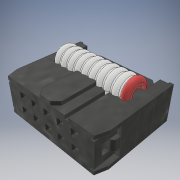
# Autodesk Inventor part: Connector-2x5
Saved by Autodesk Inventor 2018 (Build 220112000, 112)
## iProperties
Created: 2021-02-20
Part Number: Connector-2x5
Material: Všeobecné
Document SubType Name: Modeling
Designer: Jozko Mrkvicka
Density: 1 g/cm^3
Appearance: Výchozí
Author: Jozko Mrkvicka
Autodesk Inventor part; units mm, degrees
sketch "Náčrt1" plane through (0, 0, 0) normal (0, 1, 0) x (-1, 0, 0)
  line L0 (3.175, 8.89) -> (-3.175, 8.89)
  line L1 (-3.175, 8.89) -> (-3.175, -8.89)
  line L2 (-3.175, -8.89) -> (3.175, -8.89)
  line L3 (3.175, -8.89) -> (3.175, 8.89)
  line L4 (3.175, 8.89) -> (-3.175, -8.89) construction
  line L5 (-3.175, 8.89) -> (3.175, -8.89) construction
  point P0 (0, 0)
  dimension "d0" = 6.35
  dimension "d1" = 17.78
  constraints: 12 end point, 2 midpoint, 2 parallel, 1 horizontal, 1 perpendicular
  measures "d0" distance of L2.end L1.end
  measures "d1" distance of L1.end L0.end
extrude "Vysunutí1" add sketch "Náčrt1" along normal blind 15.24
sketch "Náčrt2" plane through (0, 15.24, 0) normal (0, 1, 0) x (1, 0, 0)
  line L0 (-1.5875, -6.35) -> (-1.5875, 6.35)
  line L1 (-3.175, -6.985) -> (-1.5875, -6.985)
  line L2 (-1.5875, -6.985) -> (-1.5875, 6.985)
  line L3 (-1.5875, 6.985) -> (-3.175, 6.985)
  line L4 (-3.175, 6.985) -> (-3.175, -6.985)
  line L5 (-3.175, -6.985) -> (-1.5875, 6.985) construction
  line L6 (-1.5875, -6.985) -> (-3.175, 6.985) construction
  line L7 (3.175, -6.985) -> (1.5875, -6.985)
  line L8 (1.5875, -6.985) -> (1.5875, 6.985)
  line L9 (1.5875, 6.985) -> (3.175, 6.985)
  line L10 (3.175, 6.985) -> (3.175, -6.985)
  line L11 (3.175, -6.985) -> (1.5875, 6.985) construction
  line L12 (1.5875, -6.985) -> (3.175, 6.985) construction
  point P0 (0, 0)
  point P1 (-3.175, -6.35)
  point P2 (-2.3813, 0)
  point P3 (2.3813, 0)
  dimension "d18" = 13.97
  dimension "d19" = 13.97
  constraints: 26 end point, 4 midpoint, 4 parallel, 2 horizontal, 2 perpendicular
  measures "d18" distance of L2.end L1.end
  measures "d19" distance of L7.end L8.end
extrude "Vysunutí2" cut sketch "Náčrt2" against normal blind 5.08
sketch "Náčrt3" plane through (3.175, 0, 8.89) normal (1, 0, 0) x (0, 0, -1)
  line L0 (3.81, 15.24) -> (2.54, 13.97)
  line L1 (13.97, 15.24) -> (15.24, 13.97)
  line L2 (2.54, 13.97) -> (0.635, 13.97)
  line L3 (15.24, 13.97) -> (17.145, 13.97)
  line L4 (0.635, 13.97) -> (0.635, 14.2875)
  line L5 (0.635, 14.2875) -> (0, 14.2875)
  line L6 (17.145, 13.97) -> (17.145, 14.2875)
  line L7 (17.145, 14.2875) -> (17.78, 14.2875)
  line L8 (3.81, 15.24) -> (13.97, 15.24)
  line L9 (17.78, 14.2875) -> (17.78, 16.064)
  line L10 (17.78, 16.064) -> (0, 16.064)
  line L11 (0, 16.064) -> (0, 14.2875)
  line L12 (0.635, 13.97) -> (2.54, 13.97)
  line L13 (15.24, 13.97) -> (17.145, 13.97)
  point P0 (8.89, 0)
  point P1 (8.89, 15.24)
  constraints: 28 end point, 3 parallel, 3 perpendicular, 2 horizontal
extrude "Vysunutí3" cut sketch "Náčrt3" against normal up to surface (6.35 mm away)
sketch "Náčrt4" plane through (3.175, 0, 8.89) normal (1, 0, 0) x (0, 0, -1)
  line L0 (1.905, 6.985) -> (15.875, 6.985)
  line L1 (15.875, 6.985) -> (15.875, 11.43)
  line L2 (15.875, 11.43) -> (1.905, 11.43)
  line L3 (1.905, 11.43) -> (1.905, 6.985)
  point P0 (0, 0)
  point P1 (8.89, 0)
  constraints: 8 end point, 2 parallel, 1 horizontal, 1 perpendicular
extrude "Vysunutí4" cut sketch "Náčrt4" against normal up to surface (6.35 mm away)
sketch "Náčrt5" plane through (0, 0, 0) normal (0, -1, 0) x (1, 0, 0)
  line L0 (-3.175, 6.985) -> (-3.175, -6.985) projected
  line L1 (-1.27, 5.08) -> (1.27, 5.08)
  line L2 (1.27, 5.08) -> (1.27, -5.08)
  line L3 (0.9525, 4.7625) -> (1.5875, 4.7625)
  line L4 (1.5875, 4.7625) -> (1.5875, 5.3975)
  line L5 (1.5875, 5.3975) -> (0.9525, 5.3975)
  line L6 (0.9525, 5.3975) -> (0.9525, 4.7625)
  line L7 (0.9525, 4.7625) -> (1.5875, 5.3975) construction
  line L8 (1.5875, 4.7625) -> (0.9525, 5.3975) construction
  line L9 (1.5875, 2.2225) -> (1.5875, 2.8575)
  line L10 (1.5875, 2.8575) -> (0.9525, 2.8575)
  line L11 (0.9525, 2.2225) -> (1.5875, 2.2225)
  line L12 (0.9525, 2.8575) -> (0.9525, 2.2225)
  line L13 (1.5875, -0.3175) -> (1.5875, 0.3175)
  line L14 (1.5875, 0.3175) -> (0.9525, 0.3175)
  line L15 (0.9525, -0.3175) -> (1.5875, -0.3175)
  line L16 (0.9525, 0.3175) -> (0.9525, -0.3175)
  line L17 (1.5875, -2.8575) -> (1.5875, -2.2225)
  line L18 (1.5875, -2.2225) -> (0.9525, -2.2225)
  line L19 (0.9525, -2.8575) -> (1.5875, -2.8575)
  line L20 (0.9525, -2.2225) -> (0.9525, -2.8575)
  line L21 (1.5875, -5.3975) -> (1.5875, -4.7625)
  line L22 (1.5875, -4.7625) -> (0.9525, -4.7625)
  line L23 (0.9525, -5.3975) -> (1.5875, -5.3975)
  line L24 (0.9525, -4.7625) -> (0.9525, -5.3975)
  line L25 (-0.9525, 4.7625) -> (-0.9525, 5.3975)
  line L26 (-0.9525, 5.3975) -> (-1.5875, 5.3975)
  line L27 (-1.5875, 4.7625) -> (-0.9525, 4.7625)
  line L28 (-1.5875, 5.3975) -> (-1.5875, 4.7625)
  line L29 (-0.9525, 2.2225) -> (-0.9525, 2.8575)
  line L30 (-0.9525, 2.8575) -> (-1.5875, 2.8575)
  line L31 (-1.5875, 2.2225) -> (-0.9525, 2.2225)
  line L32 (-1.5875, 2.8575) -> (-1.5875, 2.2225)
  line L33 (-0.9525, -0.3175) -> (-0.9525, 0.3175)
  line L34 (-0.9525, 0.3175) -> (-1.5875, 0.3175)
  line L35 (-1.5875, -0.3175) -> (-0.9525, -0.3175)
  line L36 (-1.5875, 0.3175) -> (-1.5875, -0.3175)
  line L37 (-0.9525, -2.8575) -> (-0.9525, -2.2225)
  line L38 (-0.9525, -2.2225) -> (-1.5875, -2.2225)
  line L39 (-1.5875, -2.8575) -> (-0.9525, -2.8575)
  line L40 (-1.5875, -2.2225) -> (-1.5875, -2.8575)
  line L41 (-0.9525, -5.3975) -> (-0.9525, -4.7625)
  line L42 (-0.9525, -4.7625) -> (-1.5875, -4.7625)
  line L43 (-1.5875, -5.3975) -> (-0.9525, -5.3975)
  line L44 (-1.5875, -4.7625) -> (-1.5875, -5.3975)
  line L45 (1.5875, -4.7625) -> (1.5875, -2.8575)
  line L46 (3.175, -3.4925) -> (2.54, -3.4925)
  line L47 (2.54, -3.4925) -> (2.54, -4.1275)
  line L48 (2.54, -4.1275) -> (3.175, -4.1275)
  line L49 (3.175, -3.4925) -> (3.175, -4.1275)
  point P0 (0, 0)
  dimension "d30" = 2.54
  dimension "d33" = 2.54
  constraints: 98 end point, 4 horizontal, 3 parallel, 3 perpendicular, 2 midpoint, 2 vertical, 72 other
  measures "d30" distance of L3.end L9.start
  measures "d33" distance of L3.end L25.start
extrude "Vysunutí5" cut sketch "Náčrt5" against normal up to surface (6.985 mm away) contours L6 L5 L4 L3 L2 L1 | L1 L2 L3 L6 | L10 L9 L11 L2 | L2 L11 L12 L10 | L14 L13 L15 L2 | L2 L15 L16 L14 | L18 L17 L19 L2 | L2 L19 L20 L18 | L22 L21 L23 L24 | L27 L28 L26 L25 | L31 L32 L30 L29 | L35 L36 L34 L33 | L39 L40 L38 L37 | L43 L44 L42 L41 | L49 L48 L47 L46
chamfer "Zkosení1" distance 0.3175 angle 45 40 edges at (1.27, 0, 5.3975) (1.27, 0, 4.7625) (0.9525, 0, 5.08) (1.5875, 0, 5.08) (1.5875, 0, 2.54) (1.27, 0, 2.2225) (0.9525, 0, 2.54) (1.27, 0, 2.8575) (1.27, 0, 0.3175) (1.27, 0, -0.3175) (1.5875, 0, 0) (0.9525, 0, 0) (1.27, 0, -2.2225) (1.5875, 0, -2.54) (0.9525, 0, -2.54) (1.27, 0, -2.8575) (1.5875, 0, -5.08) (1.27, 0, -4.7625) (0.9525, 0, -5.08) (1.27, 0, -5.3975) (-0.9525, 0, -5.08) (-1.27, 0, -5.3975) (-1.5875, 0, -5.08) (-1.27, 0, -4.7625) (-1.5875, 0, -2.54) (-1.27, 0, -2.8575) (-0.9525, 0, -2.54) (-1.27, 0, -2.2225) (-1.5875, 0, 0) (-1.27, 0, -0.3175) (-0.9525, 0, 0) (-1.27, 0, 0.3175) (-1.5875, 0, 2.54) (-1.27, 0, 2.2225) (-0.9525, 0, 2.54) (-1.27, 0, 2.8575) (-1.5875, 0, 5.08) (-1.27, 0, 4.7625) (-0.9525, 0, 5.08) (-1.27, 0, 5.3975)
sketch "Náčrt6" plane through (3.175, 0, 8.89) normal (1, 0, 0) x (0, 0, -1)
  line L0 (10.795, 0.9525) -> (10.795, 6.985)
  line L1 (10.795, 6.985) -> (6.985, 6.985)
  line L2 (6.985, 6.985) -> (6.985, 0.9525)
  line L3 (10.795, 0.9525) -> (9.8425, 0)
  line L4 (6.985, 0.9525) -> (7.9375, 0)
  line L5 (7.9375, 0) -> (9.8425, 0)
  point P0 (8.89, 0)
  constraints: 12 end point, 1 parallel
extrude "Vysunutí6" add sketch "Náčrt6" along normal blind 0.635
sketch "Náčrt7" plane through (-3.175, 0, 8.89) normal (0, 0, 1) x (1, 0, 0)
  line L0 (0.635, 0) -> (5.715, 0)
  line L1 (5.715, 0) -> (5.715, 3.81)
  line L2 (0.635, 3.81) -> (0.635, 0)
  line L3 (4.1275, 3.81) -> (4.1275, 2.54)
  line L4 (4.1275, 2.54) -> (2.2225, 2.54)
  line L5 (2.2225, 2.54) -> (2.2225, 3.81)
  line L6 (5.715, 3.81) -> (4.1275, 3.81)
  line L7 (2.2225, 3.81) -> (0.635, 3.81)
  point P0 (3.175, 0)
  point P1 (3.175, 3.81)
  constraints: 16 end point, 4 parallel, 1 horizontal, 1 perpendicular
extrude "Vysunutí7" cut sketch "Náčrt7" against normal blind 1.27
sketch "Náčrt8" plane through (3.175, 0, -8.89) normal (0, 0, -1) x (-1, 0, 0)
  line L0 (0.635, 0) -> (5.715, 0) projected
  line L1 (0.635, 3.81) -> (0.635, 0) projected
  line L2 (2.2225, 3.81) -> (0.635, 3.81) projected
  line L3 (2.2225, 2.54) -> (2.2225, 3.81) projected
  line L4 (4.1275, 2.54) -> (2.2225, 2.54) projected
  line L5 (4.1275, 3.81) -> (4.1275, 2.54) projected
  line L6 (5.715, 3.81) -> (4.1275, 3.81) projected
  line L7 (5.715, 0) -> (5.715, 3.81) projected
extrude "Vysunutí8" cut sketch "Náčrt8" against normal blind 1.27
fillet "Zaoblení1" radius 0.635 2 edges at (0, 2.54, 8.89) (0, 2.54, -8.89)
sketch "Náčrt9" plane through (-3.175, 0, 7.62) normal (0, 0, 1) x (1, 0, 0)
  line L0 (5.715, 0) -> (0.635, 0) projected
  line L1 (4.1275, 3.81) -> (5.715, 3.81) projected
  line L2 (4.1275, 2.54) -> (4.1275, 3.81) projected
  line L3 (2.2225, 2.54) -> (4.1275, 2.54) projected
  line L4 (2.2225, 3.81) -> (2.2225, 2.54) projected
  line L5 (0.635, 3.81) -> (2.2225, 3.81) projected
  line L6 (5.715, 0) -> (5.3975, 0)
  line L7 (5.3975, 0) -> (5.3975, 3.81)
  line L8 (0.635, 0) -> (0.9525, 0)
  line L9 (0.9525, 0) -> (0.9525, 3.81)
  line L10 (4.1275, 2.54) -> (2.2225, 2.54)
  line L11 (2.2225, 2.54) -> (2.2225, 1.27)
  line L12 (2.2225, 1.27) -> (4.1275, 1.27)
  line L13 (4.1275, 1.27) -> (4.1275, 2.54)
  point P0 (3.175, 0)
  dimension "d57" = 0.3175
  dimension "d58" = 0.3175
  dimension "d59" = 1.27
  constraints: 16 end point, 4 point on line, 3 perpendicular, 2 parallel, 1 horizontal
  measures "d57" distance of L0.start L6.end
  measures "d58" distance of L0.end L8.end
  measures "d59" distance of L11.end L10.end
extrude "Vysunutí9" add sketch "Náčrt9" along normal blind 0.635 contours L0 L9 L5 L4 L11 L12 L13 L2 L1 L7
ref_plane "Pracovní rovina1" through (-2.3813, 0, 7.62) normal (0, 0, 1) x (1, 0, 0)
sketch "Náčrt10" plane through (3.175, 0, -7.62) normal (0, 0, -1) x (-1, 0, 0)
  line L0 (2.2225, 2.54) -> (2.2225, 3.81) projected
  line L1 (2.2225, 2.54) -> (2.2225, 1.27) projected
  line L2 (2.2225, 1.27) -> (4.1275, 1.27) projected
  line L3 (4.1275, 1.27) -> (4.1275, 2.54) projected
  line L4 (4.1275, 3.81) -> (4.1275, 2.54) projected
  line L5 (5.3975, 3.81) -> (4.1275, 3.81) projected
  line L6 (5.3975, 3.81) -> (5.3975, 0) projected
  line L7 (5.3975, 0) -> (0.9525, 0) projected
  line L8 (0.9525, 0) -> (0.9525, 3.81) projected
  line L9 (2.2225, 3.81) -> (0.9525, 3.81) projected
  point P0 (3.175, 0)
extrude "Vysunutí10" add sketch "Náčrt10" along normal blind 0.635
ref_plane "Pracovní rovina2" through (-2.3812, 0, -7.62) normal (0, 0, -1) x (-1, 0, 0)
split_face "Rozdělit1"
split_face "Rozdělit2"
chamfer "Zkosení2" distance 1.905 distance2 0.635 1 edges at (-2.8575, 0, 8.89) measured on face at (0.3175, 10.795, 8.89)
chamfer "Zkosení3" distance 1.905 distance2 0.635 1 edges at (2.8575, 0, 8.89) measured on face at (0.3175, 10.795, 8.89)
chamfer "Zkosení4" distance 1.905 distance2 0.635 1 edges at (2.8575, 0, -8.89) measured on face at (0.3175, 10.795, -8.89)
chamfer "Zkosení5" distance 1.905 distance2 0.635 1 edges at (-2.8575, 0, -8.89) measured on face at (0.3175, 10.795, -8.89)
sketch "Náčrt11" plane through (-3.175, 13.97, -6.985) normal (0, 0, 1) x (1, 0, 0)
  line L0 (6.35, 0) -> (6.35, -6.985) projected
  line L1 (0, -12.065) -> (0, 0.3175) projected
  line L2 (6.35, -3.6512) -> (0, -3.6512)
  line L3 (0, -3.6512) -> (0, -6.0325)
  line L4 (0, -6.0325) -> (6.35, -6.0325)
  line L5 (6.35, -6.0325) -> (6.35, -3.6512)
  line L6 (6.35, -6.985) -> (0, -6.985) projected
  line L7 (4.7625, -2.54) -> (1.5875, -2.54) projected
  point P0 (3.175, -13.97)
  dimension "d94" = 0.9525
  dimension "d95" = 1.1113
  constraints: 8 end point, 2 parallel, 2 point on line, 1 horizontal, 1 perpendicular
  measures "d94" distance between parallel lines of L4 L6
  measures "d95" distance between parallel lines of L7 L2
extrude "Vysunutí11" add sketch "Náčrt11" along normal up to next contours L0 L4 L1 L2
sketch "Náčrt12" plane through (3.175, 13.97, -6.985) normal (1, 0, 0) x (0, 0, -1)
  line L0 (0, -6.985) -> (-2.8575, -6.985) projected
  line L1 (0, 0) -> (0, -3.6512) projected
  line L2 (-13.97, -6.985) -> (-13.97, -6.0325) projected
  circle A0 centre (-0.6985, -6.5098) radius 0.635
  line L3 (0, -6.985) -> (0, -6.0325)
  line L4 (0, -6.0325) -> (-13.97, -6.0325)
  line L5 (-13.97, -6.0325) -> (-13.97, -6.985)
  line L6 (0, -6.5087) -> (-13.97, -6.5087)
  circle A1 centre (-2.0955, -6.5098) radius 0.635
  circle A2 centre (-3.4925, -6.5098) radius 0.635
  circle A3 centre (-4.8895, -6.5098) radius 0.635
  circle A4 centre (-6.2865, -6.5098) radius 0.635
  circle A5 centre (-7.6835, -6.5098) radius 0.635
  circle A6 centre (-9.0805, -6.5098) radius 0.635
  circle A7 centre (-10.4775, -6.5098) radius 0.635
  circle A8 centre (-11.8745, -6.5098) radius 0.635
  circle A9 centre (-13.2715, -6.5098) radius 0.635
  circle A10 centre (-0.6985, -3.1761) radius 0.635
  circle A11 centre (-2.0955, -3.1761) radius 0.635
  circle A12 centre (-3.4925, -3.1761) radius 0.635
  circle A13 centre (-4.8895, -3.1761) radius 0.635
  circle A14 centre (-6.2865, -3.1761) radius 0.635
  circle A15 centre (-7.6835, -3.1761) radius 0.635
  circle A16 centre (-9.0805, -3.1761) radius 0.635
  circle A17 centre (-10.4775, -3.1761) radius 0.635
  circle A18 centre (-11.8745, -3.1761) radius 0.635
  circle A19 centre (-13.2715, -3.1761) radius 0.635
  line L7 (-0.6985, -6.5098) -> (-0.5398, -6.5098) construction
  line L8 (0, -6.0325) -> (-13.97, -6.0325) projected
  line L9 (-0.6985, -6.5098) -> (-0.5398, -6.5098) construction
  line L10 (-0.6985, -2.8586) -> (-13.2715, -2.8586)
  line L11 (-13.2715, -2.8586) -> (-13.2715, -3.4936)
  line L12 (-13.2715, -3.4936) -> (-0.6985, -3.4936)
  line L13 (-0.6985, -2.8586) -> (-0.6985, -3.4936)
  line L14 (-0.6985, -6.1923) -> (-13.2715, -6.1923)
  line L15 (-13.2715, -6.1923) -> (-13.2715, -6.8273)
  line L16 (-13.2715, -6.8273) -> (-0.6985, -6.8273)
  line L17 (-0.6985, -6.8273) -> (-0.6985, -6.1923)
  point P0 (-6.985, -13.97)
  dimension "d98" = 1.397
  dimension "d101" = 3.3338
  constraints: 28 end point, 20 centre point, 6 horizontal, 4 equal length, 3 vertical, 2 midpoint, 2 perpendicular, 38 other
  measures "d98" distance of L7.start A1.centre
  measures "d101" distance of L7.start A10.centre
extrude "Vysunutí12" cut sketch "Náčrt12" against normal up to surface (6.35 mm away) contours A0 L0 | L0 A0 L16 L17 L6 | L6 L17 L14 A0 L4 | A1 L0 | L0 A1 L16 | A0 L6 L17 L16 | L4 A0 | L6 A0 L14 L17 | L16 A1 L6 | L6 A1 L14 | A1 L14 L4 | L4 A1 | L16 A2 L6 | A2 L16 | L6 A2 L14 | A2 L14 L4 | L4 A2 | L16 A3 L6 | A3 L16 | L6 A3 L14 | A3 L14 L4 | L4 A3 | L16 A4 L6 | A4 L16 | L6 A4 L14 | A4 L14 L4 | L4 A4 | L16 A5 L6 | A5 L16 | L6 A5 L14 | A5 L14 L4 | L4 A5 | L16 A6 L6 | A6 L16 | L6 A6 L14 | A6 L14 L4 | L4 A6 | L16 A7 L6 | A7 L16 | L6 A7 L14 | A7 L14 L4 | L4 A7 | L16 A8 L6 | A8 L16 | L6 A8 L14 | A8 L14 L4 | L4 A8 | L16 L15 L6 A9 | A9 L6 L15 L16 | L6 L15 L14 A9 | A9 L4 L14 L15 L6 | L4 A9 | A10 L12 L13 L10 | L10 L13 L12 A10 | L10 A11 | A11 L12 L10 | A11 L12 | L10 A12 | A12 L12 L10 | A12 L12 | L10 A13 | A13 L12 L10 | A13 L12 | L10 A14 | A14 L12 L10 | A14 L12 | L10 A15 | A15 L12 L10 | A15 L12 | L10 A16 | A16 L12 L10 | A16 L12 | L10 A17 | A17 L12 L10 | A17 L12 | L10 A18 | A18 L12 L10 | A18 L12 | L10 L11 L12 A19 | A19 L12 L11 L10
extrude "Vysunutí13" cut sketch "Náčrt12" along normal up to surface (0.635 mm away) contours L16 A3 L6 | A3 L16 | L6 A3 L14 | A3 L14 L4 | L4 A3 | L16 A4 L6 | A4 L16 | L6 A4 L14 | A4 L14 L4 | L4 A4 | L16 A5 L6 | A5 L16 | L6 A5 L14 | A5 L14 L4 | L4 A5 | L16 A6 L6 | A6 L16 | L6 A6 L14 | A6 L14 L4 | L4 A6
extrude "Vysunutí14" add sketch "Náčrt12" against normal up to surface (6.35 mm away) contours A0 L0 | L0 A0 L16 L17 L6 | L6 L17 L14 A0 L4 | A1 L0 | L0 A1 L16 | L16 A1 L6 A0 | A0 L6 L17 L16 | L4 A0 | L6 A0 L14 L17 | L16 A1 L6 | L6 A1 L14 A0 | L16 A2 L6 A1 | L6 A1 L14 | A1 L14 L4 | L4 A1 | L6 A2 L14 A1 | L16 A2 L6 | A2 L16 | L6 A2 L14 | L16 A3 L6 A2 | A2 L14 L4 | L4 A2 | L6 A3 L14 A2 | L16 A3 L6 | A3 L16 | L6 A3 L14 | L16 A4 L6 A3 | A3 L14 L4 | L4 A3 | L6 A4 L14 A3 | L16 A4 L6 | A4 L16 | L6 A4 L14 | L16 A5 L6 A4 | A4 L14 L4 | L4 A4 | L6 A5 L14 A4 | L16 A5 L6 | A5 L16 | L6 A5 L14 | L16 A6 L6 A5 | A5 L14 L4 | L4 A5 | L6 A6 L14 A5 | L16 A6 L6 | A6 L16 | L6 A6 L14 | L16 A7 L6 A6 | A6 L14 L4 | L4 A6 | L6 A7 L14 A6 | L16 A7 L6 | A7 L16 | L6 A7 L14 | L16 A8 L6 A7 | A7 L14 L4 | L4 A7 | L6 A8 L14 A7 | L16 A8 L6 | A8 L16 | L6 A8 L14 | L16 A9 L6 A8 | A8 L14 L4 | L4 A8 | L6 A9 L14 A8 | L16 L15 L6 A9 | A9 L6 L15 L16 | L6 L15 L14 A9 | A9 L4 L14 L15 L6 | L4 A9 | A10 L12 L13 L10 | L10 L13 L12 A10 | A10 L12 A11 L10 | L10 A11 | A11 L12 L10 | A11 L12 | A11 L12 A12 L10 | L10 A12 | A12 L12 L10 | A12 L12 | A12 L12 A13 L10 | L10 A13 | A13 L12 L10 | A13 L12 | A13 L12 A14 L10 | L10 A14 | A14 L12 L10 | A14 L12 | A14 L12 A15 L10 | L10 A15 | A15 L12 L10 | A15 L12 | A15 L12 A16 L10 | L10 A16 | A16 L12 L10 | A16 L12 | A16 L12 A17 L10 | L10 A17 | A17 L12 L10 | A17 L12 | A17 L12 A18 L10 | L10 A18 | A18 L12 L10 | A18 L12 | A18 L12 A19 L10 | L10 L11 L12 A19 | A19 L12 L11 L10
split_face "Rozdělit3"
split_face "Rozdělit4"
split_face "Rozdělit5"
split_face "Rozdělit6"
split_face "Rozdělit7"
split_face "Rozdělit8"
split_face "Rozdělit9"
split_face "Rozdělit10"
split_face "Rozdělit11"
split_face "Rozdělit12"
split_face "Rozdělit13"
split_face "Rozdělit14"
split_face "Rozdělit15"
split_face "Rozdělit16"
split_face "Rozdělit17"
split_face "Rozdělit18"
split_face "Rozdělit19"
split_face "Rozdělit20"
split_face "Rozdělit21"
split_face "Rozdělit22"
split_face "Rozdělit23"
split_face "Rozdělit24"
split_face "Rozdělit25"
split_face "Rozdělit26"
split_face "Rozdělit27"
split_face "Rozdělit28"
split_face "Rozdělit29"
split_face "Rozdělit30"
split_face "Rozdělit31"
split_face "Rozdělit32"
split_face "Rozdělit33"
split_face "Rozdělit34"
split_face "Rozdělit35"
split_face "Rozdělit36"
split_face "Rozdělit37"
split_face "Rozdělit38"
split_face "Rozdělit39"
split_face "Rozdělit40"
split_face "Rozdělit41"
ref_plane "Pracovní rovina3" through (3.175, 6.985, 0.9525) normal (0, 1, 0) x (0, 0, 1)
split_face "Rozdělit42"
ref_plane "Pracovní rovina4" through (3.175, 10.3188, 6.985) normal (0, 1, 0) x (1, 0, 0)
split_face "Rozdělit43"
ref_plane "Pracovní rovina5" through (3.175, 6.8252, -6.2865) normal (0, 0, -1) x (-1, 0, 0)
sketch "Náčrt13" plane through (3.175, 6.8252, -6.2865) normal (0, 0, -1) x (-1, 0, 0)
  line L0 (0, 1.27) -> (0, 1.1123) projected
  line L1 (0, 0.1598) -> (0, 0) projected
  line L2 (0, 1.27) -> (0, 0)
  line L3 (0, 3.3338) -> (0, 3.4936) projected
  line L4 (0, 3.4936) -> (0, 4.6037) projected
  line L5 (0, 3.3338) -> (0, 4.6037)
  arc A0 (0.4793, 3.9688) -> (0, 0.635) centre (0.0371, 2.331) ccw
  point P0 (3.175, -6.8252)
  point P1 (0, 4.2862)
  constraints: 4 end point, 2 point on circle, 2 vertical, 1 centre point, 1 midpoint
sweep "Tažení2" add profiles "Náčrt12" path "Náčrt13" path curves A0 contours A0 L0 | L0 A0 L16 L17 L6 | L6 A0 L4 L3 | L6 L17 L14 A0 L4 | A1 L0 | L0 A1 L16 | L16 A1 L6 A0 | A0 L6 L17 L16 | L4 A0 | L6 A0 L14 L17 | L16 A1 L6 | L6 A1 L14 A0 | A0 L14 A1 L4 | L16 A2 L6 A1 | L6 A1 L14 | A1 L14 L4 | L4 A1 | L6 A2 L14 A1 | L16 A2 L6 | A2 L16 | A1 L14 A2 L4 | L6 A2 L14 | L16 A3 L6 A2 | A2 L14 L4 | L4 A2 | L6 A3 L14 A2 | L16 A3 L6 | A3 L16 | A2 L14 A3 L4 | L6 A3 L14 | L16 A4 L6 A3 | A3 L14 L4 | L4 A3 | L6 A4 L14 A3 | L16 A4 L6 | A4 L16 | A3 L14 A4 L4 | L6 A4 L14 | L16 A5 L6 A4 | A4 L14 L4 | L4 A4 | L6 A5 L14 A4 | L16 A5 L6 | A5 L16 | A4 L14 A5 L4 | L6 A5 L14 | L16 A6 L6 A5 | A5 L14 L4 | L4 A5 | L6 A6 L14 A5 | L16 A6 L6 | A6 L16 | A5 L14 A6 L4 | L6 A6 L14 | L16 A7 L6 A6 | A6 L14 L4 | L4 A6 | L6 A7 L14 A6 | L16 A7 L6 | A7 L16 | A6 L14 A7 L4 | L6 A7 L14 | L16 A8 L6 A7 | A7 L14 L4 | L4 A7 | L6 A8 L14 A7 | L16 A8 L6 | A8 L16 | A7 L14 A8 L4 | L6 A8 L14 | L16 A9 L6 A8 | A8 L14 L4 | L4 A8 | L6 A9 L14 A8 | L16 L15 L6 A9 | A9 L6 L15 L16 | A8 L14 A9 L4 | L6 L15 L14 A9 | A9 L4 L14 L15 L6 | L6 L2 L4 A9 | L4 A9
ref_plane "Pracovní rovina6" through (-1.7463, 3.81, -8.89) normal (0, -1, 0) x (1, 0, 0)
split_face "Rozdělit44"
